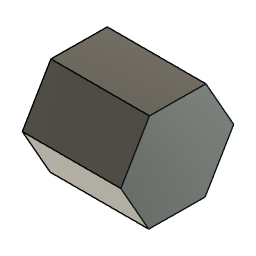
Container Beans - Shell - No Bottom v1.0 v1 (Autodesk Fusion 360 design; units mm, degrees)
Autodesk Fusion 360 part; units mm, degrees
sketch "Sketch1" plane through (0, 0, 0) normal (1, 0, 0) x (0, 1, 0)
  line L0 (174.7205, 297.2802) -> (-170.0919, 299.9525)
  line L1 (-170.0919, 299.9525) -> (-344.8124, 2.6723)
  line L2 (-344.8124, 2.6723) -> (-174.7205, -297.2802)
  line L3 (-174.7205, -297.2802) -> (170.0919, -299.9525)
  line L4 (170.0919, -299.9525) -> (344.8124, -2.6723)
  line L5 (344.8124, -2.6723) -> (174.7205, 297.2802)
  line L6 (84.6545, -149.2858) -> (171.6126, -1.33)
  line L7 (171.6126, -1.33) -> (86.9581, 147.9558)
  line L8 (86.9581, 147.9558) -> (-84.6545, 149.2858)
  line L9 (-84.6545, 149.2858) -> (-171.6126, 1.33)
  line L10 (-171.6126, 1.33) -> (-86.9581, -147.9558)
  line L11 (-86.9581, -147.9558) -> (84.6545, -149.2858)
  dimension "d1" = -150
extrude "Extrude1" add sketch "Sketch1" along normal blind 300 contours L6 L7 L8 L9 L10 L11
sketch "Sketch2" plane through (0, 0, 0) normal (-1, 0, 0) x (0, -1, 0)
  line L0 (-84.6545, -149.2858) -> (86.9581, -147.9558)
  line L1 (86.9581, -147.9558) -> (171.6126, 1.33)
  line L2 (171.6126, 1.33) -> (84.6545, 149.2858)
  line L3 (84.6545, 149.2858) -> (-86.9581, 147.9558)
  line L4 (-86.9581, 147.9558) -> (-171.6126, -1.33)
  line L5 (-171.6126, -1.33) -> (-84.6545, -149.2858)
  line L6 (174.7205, -297.2802) -> (344.8124, 2.6723)
  line L7 (344.8124, 2.6723) -> (170.0919, 299.9525)
  line L8 (170.0919, 299.9525) -> (-174.7205, 297.2802)
  line L9 (-174.7205, 297.2802) -> (-344.8124, -2.6723)
  line L10 (-344.8124, -2.6723) -> (-170.0919, -299.9525)
  line L11 (-170.0919, -299.9525) -> (174.7205, -297.2802)
sketch "Sketch3" plane through (300, 0, 0) normal (1, 0, 0) x (0, 1, 0)
  line L0 (-86.9581, -147.9558) -> (84.6545, -149.2858)
  line L1 (84.6545, -149.2858) -> (171.6126, -1.33)
  line L2 (171.6126, -1.33) -> (86.9581, 147.9558)
  line L3 (86.9581, 147.9558) -> (-84.6545, 149.2858)
  line L4 (-84.6545, 149.2858) -> (-171.6126, 1.33)
  line L5 (-171.6126, 1.33) -> (-86.9581, -147.9558)
